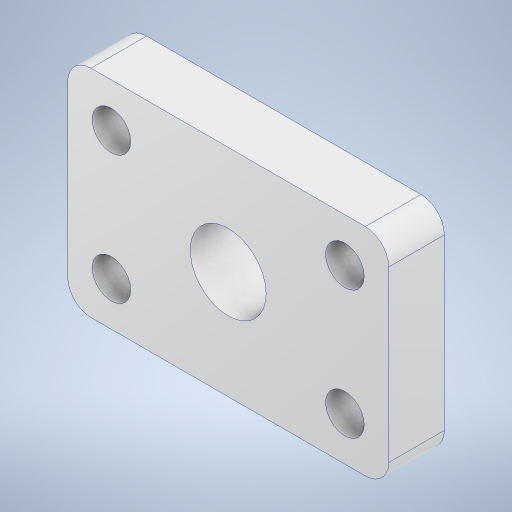
# Autodesk Inventor part: Printhead Belt Retainer Top Spacer
Saved by Autodesk Inventor 2024 (Build 280153000, 153)
## iProperties
Created: 2025-01-04
Part Number: Printhead Belt Retainer Top Spacer
Material: Aluminum 6061
Document SubType Name: Modeling
Designer: Ishaan
Density: 2.7 g/cm^3
Appearance: Aluminum - Flat
Author: Ishaan
Autodesk Inventor part; units mm, degrees
ref_plane "YZ Plane" through (0, 0, 0) normal (1, 0, 0) x (0, 1, 0)
ref_plane "XZ Plane" through (0, 0, 0) normal (0, 1, 0) x (-1, 0, 0)
ref_plane "XY Plane" through (0, 0, 0) normal (0, 0, 1) x (1, 0, 0)
sketch "Sketch1" plane through (0, 0, 0) normal (0, 0, 1) x (1, 0, 0)
  line L0 (13.75, -9.25) -> (-13.75, -9.25)
  line L1 (-13.75, -9.25) -> (-13.75, 9.25)
  line L2 (-13.75, 9.25) -> (13.75, 9.25)
  line L3 (13.75, 9.25) -> (13.75, -9.25)
  line L4 (13.75, -9.25) -> (-13.75, 9.25) construction
  line L5 (-13.75, -9.25) -> (13.75, 9.25) construction
  point P0 (0, 0)
  dimension "d0" = 27.5
  dimension "d1" = 18.5
  constraints: 12 end point, 2 midpoint, 2 parallel, 1 horizontal, 1 perpendicular
  measures "d0" distance of L1.end L2.end
  measures "d1" distance of L0.end L1.end
extrude "Extrusion1" add sketch "Sketch1" along normal blind 4.7625
sketch "Sketch2" plane through (0, 0, 4.7625) normal (0, 0, 1) x (1, 0, 0)
  line L0 (10, -5.5) -> (-10, -5.5) construction
  line L1 (-10, -5.5) -> (-10, 5.5) construction
  line L2 (-10, 5.5) -> (10, 5.5) construction
  line L3 (10, 5.5) -> (10, -5.5) construction
  line L4 (10, -5.5) -> (-10, 5.5) construction
  line L5 (-10, -5.5) -> (10, 5.5) construction
  point P0 (0, 0)
  dimension "d4" = 20
  dimension "d5" = 11
  constraints: 12 end point, 2 midpoint, 2 parallel, 1 horizontal, 1 perpendicular
  measures "d4" distance of L1.end L2.end
  measures "d5" distance of L0.end L1.end
hole "Hole1" at (-10, 5.5, 4.7625) at (10, 5.5, 4.7625) at (10, -5.5, 4.7625) at (-10, -5.5, 4.7625) direction (0, 0, -1) diameter 3.3 end through all
sketch "Sketch3" plane through (0, 0, 4.7625) normal (0, 0, 1) x (1, 0, 0)
  point P0 (0, 0)
hole "Hole2" at (0, 0, 4.7625) direction (0, 0, -1) diameter 6.5 end through all
fillet "Fillet1" radius 2 4 edges at (-13.75, 9.25, 2.3813) (-13.75, -9.25, 2.3813) (13.75, -9.25, 2.3813) (13.75, 9.25, 2.3813)
body "Solid1"
